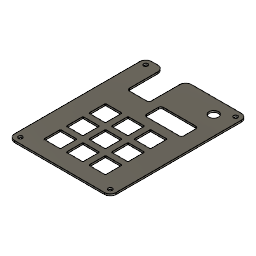
Case_Upper (Autodesk Fusion 360 design; units mm, degrees)
part number: 2026-01-01-12-40-00-996
Autodesk Fusion 360 part; units mm, degrees
sketch "ModuPad_Upper-Plate-2025-12-28T20_50_54.815Z" plane through (0, 0, 0) normal (0, 0, 1) x (1, 0, 0)
  line L0 (5.8588, 55.5041) -> (18.8588, 55.5041)
  line L1 (5.8588, 41.5041) -> (18.8588, 41.5041)
  line L2 (5.3588, 55.0041) -> (5.3588, 42.0041)
  line L3 (19.3588, 55.0041) -> (19.3588, 42.0041)
  arc A0 (5.8588, 55.5041) -> (5.3588, 55.0041) centre (5.8588, 55.0041) ccw
  arc A1 (19.3588, 55.0041) -> (18.8588, 55.5041) centre (18.8588, 55.0041) ccw
  arc A2 (5.3588, 42.0041) -> (5.8588, 41.5041) centre (5.8588, 42.0041) ccw
  arc A3 (18.8588, 41.5041) -> (19.3588, 42.0041) centre (18.8588, 42.0041) ccw
  line L4 (24.9088, 55.5041) -> (37.9088, 55.5041)
  line L5 (24.9088, 41.5041) -> (37.9088, 41.5041)
  line L6 (24.4088, 55.0041) -> (24.4088, 42.0041)
  line L7 (38.4088, 55.0041) -> (38.4088, 42.0041)
  arc A4 (24.9088, 55.5041) -> (24.4088, 55.0041) centre (24.9088, 55.0041) ccw
  arc A5 (38.4088, 55.0041) -> (37.9088, 55.5041) centre (37.9088, 55.0041) ccw
  arc A6 (24.4088, 42.0041) -> (24.9088, 41.5041) centre (24.9088, 42.0041) ccw
  arc A7 (37.9088, 41.5041) -> (38.4088, 42.0041) centre (37.9088, 42.0041) ccw
  line L8 (43.9588, 55.5041) -> (56.9588, 55.5041)
  line L9 (43.9588, 41.5041) -> (56.9588, 41.5041)
  line L10 (43.4588, 55.0041) -> (43.4588, 42.0041)
  line L11 (57.4588, 55.0041) -> (57.4588, 42.0041)
  arc A8 (43.9588, 55.5041) -> (43.4588, 55.0041) centre (43.9588, 55.0041) ccw
  arc A9 (57.4588, 55.0041) -> (56.9588, 55.5041) centre (56.9588, 55.0041) ccw
  arc A10 (43.4588, 42.0041) -> (43.9588, 41.5041) centre (43.9588, 42.0041) ccw
  arc A11 (56.9588, 41.5041) -> (57.4588, 42.0041) centre (56.9588, 42.0041) ccw
  line L12 (5.8588, 36.4541) -> (18.8588, 36.4541)
  line L13 (5.8588, 22.4541) -> (18.8588, 22.4541)
  line L14 (5.3588, 35.9541) -> (5.3588, 22.9541)
  line L15 (19.3588, 35.9541) -> (19.3588, 22.9541)
  arc A12 (5.8588, 36.4541) -> (5.3588, 35.9541) centre (5.8588, 35.9541) ccw
  arc A13 (19.3588, 35.9541) -> (18.8588, 36.4541) centre (18.8588, 35.9541) ccw
  arc A14 (5.3588, 22.9541) -> (5.8588, 22.4541) centre (5.8588, 22.9541) ccw
  arc A15 (18.8588, 22.4541) -> (19.3588, 22.9541) centre (18.8588, 22.9541) ccw
  line L16 (24.9088, 36.4541) -> (37.9088, 36.4541)
  line L17 (24.9088, 22.4541) -> (37.9088, 22.4541)
  line L18 (24.4088, 35.9541) -> (24.4088, 22.9541)
  line L19 (38.4088, 35.9541) -> (38.4088, 22.9541)
  arc A16 (24.9088, 36.4541) -> (24.4088, 35.9541) centre (24.9088, 35.9541) ccw
  arc A17 (38.4088, 35.9541) -> (37.9088, 36.4541) centre (37.9088, 35.9541) ccw
  arc A18 (24.4088, 22.9541) -> (24.9088, 22.4541) centre (24.9088, 22.9541) ccw
  arc A19 (37.9088, 22.4541) -> (38.4088, 22.9541) centre (37.9088, 22.9541) ccw
  line L20 (43.9588, 36.4541) -> (56.9588, 36.4541)
  line L21 (43.9588, 22.4541) -> (56.9588, 22.4541)
  line L22 (43.4588, 35.9541) -> (43.4588, 22.9541)
  line L23 (57.4588, 35.9541) -> (57.4588, 22.9541)
  arc A20 (43.9588, 36.4541) -> (43.4588, 35.9541) centre (43.9588, 35.9541) ccw
  arc A21 (57.4588, 35.9541) -> (56.9588, 36.4541) centre (56.9588, 35.9541) ccw
  arc A22 (43.4588, 22.9541) -> (43.9588, 22.4541) centre (43.9588, 22.9541) ccw
  arc A23 (56.9588, 22.4541) -> (57.4588, 22.9541) centre (56.9588, 22.9541) ccw
  line L24 (5.8588, 17.4041) -> (18.8588, 17.4041)
  line L25 (5.8588, 3.4041) -> (18.8588, 3.4041)
  line L26 (5.3588, 16.9041) -> (5.3588, 3.9041)
  line L27 (19.3588, 16.9041) -> (19.3588, 3.9041)
  arc A24 (5.8588, 17.4041) -> (5.3588, 16.9041) centre (5.8588, 16.9041) ccw
  arc A25 (19.3588, 16.9041) -> (18.8588, 17.4041) centre (18.8588, 16.9041) ccw
  arc A26 (5.3588, 3.9041) -> (5.8588, 3.4041) centre (5.8588, 3.9041) ccw
  arc A27 (18.8588, 3.4041) -> (19.3588, 3.9041) centre (18.8588, 3.9041) ccw
  line L28 (24.9088, 17.4041) -> (37.9088, 17.4041)
  line L29 (24.9088, 3.4041) -> (37.9088, 3.4041)
  line L30 (24.4088, 16.9041) -> (24.4088, 3.9041)
  line L31 (38.4088, 16.9041) -> (38.4088, 3.9041)
  arc A28 (24.9088, 17.4041) -> (24.4088, 16.9041) centre (24.9088, 16.9041) ccw
  arc A29 (38.4088, 16.9041) -> (37.9088, 17.4041) centre (37.9088, 16.9041) ccw
  arc A30 (24.4088, 3.9041) -> (24.9088, 3.4041) centre (24.9088, 3.9041) ccw
  arc A31 (37.9088, 3.4041) -> (38.4088, 3.9041) centre (37.9088, 3.9041) ccw
  line L32 (43.9588, 17.4041) -> (56.9588, 17.4041)
  line L33 (43.9588, 3.4041) -> (56.9588, 3.4041)
  line L34 (43.4588, 16.9041) -> (43.4588, 3.9041)
  line L35 (57.4588, 16.9041) -> (57.4588, 3.9041)
  arc A32 (43.9588, 17.4041) -> (43.4588, 16.9041) centre (43.9588, 16.9041) ccw
  arc A33 (57.4588, 16.9041) -> (56.9588, 17.4041) centre (56.9588, 16.9041) ccw
  arc A34 (43.4588, 3.9041) -> (43.9588, 3.4041) centre (43.9588, 3.9041) ccw
  arc A35 (56.9588, 3.4041) -> (57.4588, 3.9041) centre (56.9588, 3.9041) ccw
  line L36 (-10.9412, -10.0959) -> (75.0588, -10.0959)
  line L37 (75.0588, -10.0959) -> (75.0588, 105.9041)
  line L38 (75.0588, 105.9041) -> (-10.9412, 105.9041)
  line L39 (-10.9412, 105.9041) -> (-10.9412, -10.0959)
  line L40 (4.3088, 105.9041) -> (22.8088, 105.9041)
  line L41 (22.8088, 105.9041) -> (22.8088, 74.9041)
  line L42 (22.8088, 74.9041) -> (4.3088, 74.9041)
  line L43 (4.3088, 74.9041) -> (4.3088, 105.9041)
  circle A36 centre (-5.9412, 100.9041) radius 1.7
  circle A37 centre (70.0588, 100.9041) radius 1.7
  circle A38 centre (70.0588, -5.0959) radius 1.7
  circle A39 centre (-5.9412, -5.0959) radius 1.7
  line L44 (30.5588, 77.1541) -> (62.0588, 77.1541)
  line L45 (62.0588, 77.1541) -> (62.0588, 63.1541)
  line L46 (62.0588, 63.1541) -> (30.5588, 63.1541)
  line L47 (30.5588, 63.1541) -> (30.5588, 77.1541)
  circle A40 centre (59.0588, 93.4041) radius 4
  dimension "d1" = 86
  dimension "d2" = 116
  dimension "d3" = 16.3
  dimension "d4" = 13.5
  dimension "d5" = 18.5
  dimension "d6" = 31
  dimension "d7" = 15.25
  dimension "d8" = 3.4
  dimension "d9" = 5
  dimension "d10" = 5
  dimension "d11" = 3.4
  dimension "d12" = 5
  dimension "d13" = 5
  dimension "d14" = 3.4
  dimension "d15" = 5
  dimension "d16" = 5
  dimension "d17" = 3.4
  dimension "d18" = 5
  dimension "d19" = 5
  dimension "d20" = 31.5
  dimension "d21" = 14
  dimension "d22" = 13
  dimension "d23" = 28.75
  dimension "d24" = 8
  dimension "d25" = 12.5
  dimension "d26" = 16
  constraint horizontal L36
  constraint vertical L37
  constraint horizontal L38
  constraint vertical L39
  constraint horizontal L40
  constraint vertical L41
  constraint horizontal L42
  constraint vertical L43
  constraint coincident L38 L40.start
  constraint horizontal L44
  constraint vertical L45
  constraint horizontal L46
  constraint vertical L47
  measures "d1" distance of L36.start L36.end
  measures "d2" distance of L36.start L38.end
  measures "d3" distance of L26 L39
  measures "d4" distance of L25 L36
  measures "d5" distance of L40.start L40.end
  measures "d6" distance of L40.start L42.end
  measures "d7" distance of L39 L43
  measures "d8" diameter of A36
  measures "d9" distance of L38 A36.centre
  measures "d10" distance of L39 A36.centre
  measures "d11" diameter of A37
  measures "d12" distance of L38 A37.centre
  measures "d13" distance of L37 A37.centre
  measures "d14" diameter of A38
  measures "d15" distance of L37 A38.centre
  measures "d16" distance of L36 A38.centre
  measures "d17" diameter of A39
  measures "d18" distance of L36 A39.centre
  measures "d19" distance of L39 A39.centre
  measures "d20" distance of L44.start L44.end
  measures "d21" distance of L44.start L46.end
  measures "d22" distance of L37 L45
  measures "d23" distance of L38 L44
  measures "d24" diameter of A40
  measures "d25" distance of L38 A40.centre
  measures "d26" distance of L37 A40.centre
extrude "Extrude1" add sketch "ModuPad_Upper-Plate-2025-12-28T20_50_54.815Z" along normal blind 1.5 contours L36 L37 L38 L39 L41 L42 L43
fillet "Fillet1" radius 5 6 edges at (75.0588, 105.9041, 0.75) (-10.9412, -10.0959, 0.75) (75.0588, -10.0959, 0.75) (-10.9412, 105.9041, 0.75) (4.3088, 105.9041, 0.75) (22.8088, 105.9041, 0.75)
fillet "Fillet2" radius 2 4 edges at (30.5588, 63.1541, 0.75) (62.0588, 63.1541, 0.75) (30.5588, 77.1541, 0.75) (62.0588, 77.1541, 0.75)
fillet "Fillet3" radius 2 2 edges at (22.8088, 74.9041, 0.75) (4.3088, 74.9041, 0.75)
